Autodesk Fusion 360 part; units mm, degrees
(part 2 of 6)
  spline S358 degree 3 poles (-36.8879, 6.0923) (-36.784, 6.1608) (-36.7137, 6.2296) (-36.6303, 6.3216) knots 0 0 0 0 1 1 1 1
  spline S359 degree 3 poles (-36.6303, 6.3216) (-35.9723, 7.0157) (-35.2211, 7.6265) (-34.5007, 8.2547) knots 0 0 0 0 1 1 1 1
  spline S360 degree 3 poles (-34.5007, 8.2547) (-33.785, 8.879) (-33.0973, 9.5191) (-32.4627, 10.2268) knots 0 0 0 0 1 1 1 1
  spline S361 degree 3 poles (-32.4627, 10.2268) (-32.4451, 10.2088) (-32.4274, 10.1908) (-32.4092, 10.1722) knots 0 0 0 0 1 1 1 1
  spline S362 degree 3 poles (-32.4092, 10.1722) (-32.0575, 9.8145) (-31.7032, 9.4616) (-31.3264, 9.1303) knots 0 0 0 0 1 1 1 1
  spline S363 degree 3 poles (-31.3264, 9.1303) (-31.1837, 9.0046) (-31.0471, 8.8776) (-30.9171, 8.7388) knots 0 0 0 0 1 1 1 1
  spline S364 degree 3 poles (-30.9171, 8.7388) (-30.5101, 8.3132) (-30.1527, 8.1968) (-29.574, 8.1338) knots 0 0 0 0 1 1 1 1
  spline S365 degree 3 poles (-29.574, 8.1338) (-29.5084, 8.1252) (-29.4428, 8.1165) (-29.3772, 8.1077) knots 0 0 0 0 1 1 1 1
  spline S366 degree 3 poles (-29.3772, 8.1077) (-28.6438, 8.0188) (-27.9174, 8.0735) (-27.1848, 8.142) knots 0 0 0 0 1 1 1 1
  spline S367 degree 3 poles (-27.1848, 8.142) (-27.0333, 8.1561) (-26.8818, 8.17) (-26.7303, 8.1834) knots 0 0 0 0 1 1 1 1
  spline S368 degree 3 poles (-26.7303, 8.1834) (-26.6934, 8.1868) (-26.6565, 8.1901) (-26.6185, 8.1935) knots 0 0 0 0 1 1 1 1
  spline S369 degree 3 poles (-26.6185, 8.1935) (-26.3222, 8.2187) (-26.0268, 8.2275) (-25.7295, 8.224) knots 0 0 0 0 1 1 1 1
  spline S370 degree 3 poles (-25.7295, 8.224) (-25.4397, 8.2252) (-25.2695, 8.3218) (-25.0565, 8.5173) knots 0 0 0 0 1 1 1 1
  spline S371 degree 3 poles (-25.0565, 8.5173) (-24.9242, 8.5999) (-24.8512, 8.6377) (-24.6958, 8.6532) knots 0 0 0 0 1 1 1 1
  spline S372 degree 3 poles (-24.6958, 8.6532) (-24.4841, 8.7055) (-24.3698, 8.8291) (-24.2316, 8.9932) knots 0 0 0 0 1 1 1 1
  spline S373 degree 3 poles (-24.2316, 8.9932) (-24.1195, 9.1809) (-24.1288, 9.3727) (-24.1703, 9.5823) knots 0 0 0 0 1 1 1 1
  spline S374 degree 3 poles (-24.1703, 9.5823) (-24.2817, 9.9169) (-24.5269, 10.198) (-24.7398, 10.4737) knots 0 0 0 0 1 1 1 1
  spline S375 degree 3 poles (-24.7398, 10.4737) (-24.7778, 10.5239) (-24.8146, 10.5749) (-24.8506, 10.6265) knots 0 0 0 0 1 1 1 1
  spline S376 degree 3 poles (-24.8506, 10.6265) (-25.0198, 10.8677) (-25.0198, 10.8677) (-25.1822, 10.9142) knots 0 0 0 0 1 1 1 1
  spline S377 degree 3 poles (-25.1822, 10.9142) (-25.4781, 11.0159) (-25.7069, 11.2146) (-25.9398, 11.4183) knots 0 0 0 0 1 1 1 1
  spline S378 degree 3 poles (-25.9398, 11.4183) (-25.5444, 11.2634) (-25.1618, 11.083) (-24.7776, 10.9027) knots 0 0 0 0 1 1 1 1
  spline S379 degree 3 poles (-24.7776, 10.9027) (-24.4919, 10.7687) (-24.2046, 10.638) (-23.9172, 10.5075) knots 0 0 0 0 1 1 1 1
  spline S380 degree 3 poles (-23.9172, 10.5075) (-23.8009, 10.4547) (-23.6847, 10.4016) (-23.5685, 10.3486) knots 0 0 0 0 1 1 1 1
  spline S381 degree 3 poles (-23.5685, 10.3486) (-23.3419, 10.2452) (-23.1153, 10.142) (-22.8884, 10.0394) knots 0 0 0 0 1 1 1 1
  spline S382 degree 3 poles (-22.8884, 10.0394) (-22.8505, 10.0223) (-22.8126, 10.0051) (-22.7735, 9.9874) knots 0 0 0 0 1 1 1 1
  spline S383 degree 3 poles (-22.7735, 9.9874) (-22.7002, 9.9543) (-22.627, 9.9212) (-22.5537, 9.8881) knots 0 0 0 0 1 1 1 1
  spline S384 degree 3 poles (-22.5537, 9.8881) (-22.503, 9.8652) (-22.503, 9.8652) (-22.4513, 9.8418) knots 0 0 0 0 1 1 1 1
  spline S385 degree 3 poles (-22.4513, 9.8418) (-22.4218, 9.8285) (-22.3923, 9.8152) (-22.3619, 9.8015) knots 0 0 0 0 1 1 1 1
  spline S386 degree 3 poles (-22.3619, 9.8015) (-22.3034, 9.7745) (-22.2453, 9.7467) (-22.1885, 9.7163) knots 0 0 0 0 1 1 1 1
  spline S387 degree 3 poles (-22.1885, 9.7163) (-21.9936, 9.6149) (-21.8307, 9.5775) (-21.6123, 9.5674) knots 0 0 0 0 1 1 1 1
  spline S388 degree 3 poles (-21.6123, 9.5674) (-21.5658, 9.5644) (-21.5658, 9.5644) (-21.5185, 9.5615) knots 0 0 0 0 1 1 1 1
  spline S389 degree 3 poles (-21.5185, 9.5615) (-21.4183, 9.5554) (-21.3182, 9.5503) (-21.218, 9.5452) knots 0 0 0 0 1 1 1 1
  spline S390 degree 3 poles (-21.218, 9.5452) (-21.1484, 9.5413) (-21.0788, 9.5374) (-21.0092, 9.5334) knots 0 0 0 0 1 1 1 1
  spline S391 degree 3 poles (-21.0092, 9.5334) (-20.4466, 9.5024) (-19.8842, 9.482) (-19.3206, 9.4874) knots 0 0 0 0 1 1 1 1
  spline S392 degree 3 poles (-19.3206, 9.4874) (-19.2891, 9.4876) (-19.2575, 9.4878) (-19.225, 9.488) knots 0 0 0 0 1 1 1 1
  spline S393 degree 3 poles (-19.225, 9.488) (-18.1292, 9.5018) (-16.7384, 9.7508) (-15.913, 10.5426) knots 0 0 0 0 1 1 1 1
  spline S394 degree 3 poles (-15.913, 10.5426) (-15.7382, 10.7656) (-15.6089, 11.0119) (-15.6224, 11.3025) knots 0 0 0 0 1 1 1 1
  spline S395 degree 3 poles (-15.6224, 11.3025) (-15.6863, 11.7846) (-16.0023, 12.0234) (-16.3668, 12.3103) knots 0 0 0 0 1 1 1 1
  spline S396 degree 3 poles (-16.3668, 12.3103) (-16.8909, 12.6992) (-17.4415, 12.8815) (-18.0684, 13.0434) knots 0 0 0 0 1 1 1 1
  spline S397 degree 3 poles (-18.0684, 13.0434) (-18.3707, 13.1253) (-18.6252, 13.2381) (-18.8935, 13.3979) knots 0 0 0 0 1 1 1 1
  spline S398 degree 3 poles (-18.8935, 13.3979) (-19.3521, 13.6695) (-19.8084, 13.7489) (-20.3289, 13.6199) knots 0 0 0 0 1 1 1 1
  spline S399 degree 3 poles (-20.3289, 13.6199) (-20.5709, 13.5372) (-20.7719, 13.3642) (-20.9673, 13.2038) knots 0 0 0 0 1 1 1 1
  spline S400 degree 3 poles (-20.9673, 13.2038) (-21.0003, 13.2287) (-21.0003, 13.2287) (-21.034, 13.2542) knots 0 0 0 0 1 1 1 1
  spline S401 degree 3 poles (-21.034, 13.2542) (-21.681, 13.7272) (-22.4516, 13.9242) (-23.232, 14.051) knots 0 0 0 0 1 1 1 1
  spline S402 degree 3 poles (-23.232, 14.051) (-23.9763, 14.1741) (-24.6236, 14.5053) (-25.27, 14.8822) knots 0 0 0 0 1 1 1 1
  spline S403 degree 3 poles (-25.27, 14.8822) (-25.294, 14.896) (-25.3179, 14.9098) (-25.3425, 14.9239) knots 0 0 0 0 1 1 1 1
  spline S404 degree 3 poles (-25.3425, 14.9239) (-25.9243, 15.2588) (-26.4859, 15.6239) (-27.0332, 16.0126) knots 0 0 0 0 1 1 1 1
  spline S405 degree 3 poles (-27.0332, 16.0126) (-27.1228, 16.0743) (-27.2132, 16.1308) (-27.3071, 16.1857) knots 0 0 0 0 1 1 1 1
  spline S406 degree 3 poles (-27.3071, 16.1857) (-27.4896, 16.2931) (-27.661, 16.4146) (-27.8337, 16.5369) knots 0 0 0 0 1 1 1 1
  spline S407 degree 3 poles (-27.8337, 16.5369) (-28.0321, 16.6772) (-28.2298, 16.8138) (-28.4401, 16.9359) knots 0 0 0 0 1 1 1 1
  spline S408 degree 3 poles (-28.4401, 16.9359) (-28.5356, 16.993) (-28.6281, 17.0538) (-28.7209, 17.1152) knots 0 0 0 0 1 1 1 1
  spline S409 degree 3 poles (-28.7209, 17.1152) (-29.3537, 17.5298) (-30.124, 18.008) (-30.9074, 17.8632) knots 0 0 0 0 1 1 1 1
  spline S410 degree 3 poles (-30.9074, 17.8632) (-31.0398, 17.8256) (-31.1407, 17.7437) (-31.2552, 17.6685) knots 0 0 0 0 1 1 1 1
  spline S411 degree 3 poles (-31.2552, 17.6685) (-31.3254, 17.648) (-31.3962, 17.6296) (-31.4674, 17.613) knots 0 0 0 0 1 1 1 1
  spline S412 degree 3 poles (-31.4674, 17.613) (-31.8172, 17.5249) (-32.0335, 17.3244) (-32.2801, 17.0698) knots 0 0 0 0 1 1 1 1
  spline S413 degree 3 poles (-32.2801, 17.0698) (-32.3791, 16.9688) (-32.481, 16.8718) (-32.5848, 16.7757) knots 0 0 0 0 1 1 1 1
  spline S414 degree 3 poles (-32.5848, 16.7757) (-32.617, 16.7458) (-32.6492, 16.7159) (-32.6824, 16.685) knots 0 0 0 0 1 1 1 1
  spline S415 degree 3 poles (-32.6824, 16.685) (-32.7566, 16.6121) (-32.7566, 16.6121) (-32.8436, 16.6035) knots 0 0 0 0 1 1 1 1
  spline S416 degree 3 poles (-32.8436, 16.6035) (-32.8609, 16.6312) (-32.8782, 16.6588) (-32.896, 16.6872) knots 0 0 0 0 1 1 1 1
  spline S417 degree 3 poles (-32.896, 16.6872) (-33.2135, 17.1932) (-33.534, 17.6965) (-33.8742, 18.1877) knots 0 0 0 0 1 1 1 1
  spline S418 degree 3 poles (-33.8742, 18.1877) (-33.8992, 18.2239) (-33.9241, 18.2601) (-33.9498, 18.2975) knots 0 0 0 0 1 1 1 1
  spline S419 degree 3 poles (-33.9498, 18.2975) (-34.064, 18.4608) (-34.1797, 18.6215) (-34.3055, 18.7762) knots 0 0 0 0 1 1 1 1
  spline S420 degree 3 poles (-34.3055, 18.7762) (-34.6205, 19.1647) (-34.8641, 19.5705) (-35.0993, 20.0112) knots 0 0 0 0 1 1 1 1
  spline S421 degree 3 poles (-35.0993, 20.0112) (-35.5267, 20.8108) (-36.0105, 21.6081) (-36.9172, 21.9228) knots 0 0 0 0 1 1 1 1
  spline S422 degree 3 poles (-36.9172, 21.9228) (-37.0913, 21.9594) (-37.2565, 21.9237) (-37.4289, 21.8904) knots 0 0 0 0 1 1 1 1
  spline S423 degree 3 poles (-37.4289, 21.8904) (-37.4678, 21.8831) (-37.5066, 21.8758) (-37.5466, 21.8683) knots 0 0 0 0 1 1 1 1
  spline S424 degree 3 poles (-37.5466, 21.8683) (-38.3823, 21.6952) (-38.9884, 21.1445) (-39.5214, 20.5068) knots 0 0 0 0 1 1 1 1
  spline S425 degree 3 poles (-39.5214, 20.5068) (-39.5486, 20.4751) (-39.5758, 20.4434) (-39.6038, 20.4107) knots 0 0 0 0 1 1 1 1
  spline S426 degree 3 poles (-39.6038, 20.4107) (-39.7638, 20.2192) (-39.8932, 20.0166) (-40.0164, 19.8) knots 0 0 0 0 1 1 1 1
  spline S427 degree 3 poles (-40.0164, 19.8) (-40.0388, 19.7605) (-40.0612, 19.7211) (-40.0844, 19.6805) knots 0 0 0 0 1 1 1 1
  spline S428 degree 3 poles (-40.0844, 19.6805) (-40.1778, 19.515) (-40.2706, 19.3492) (-40.3602, 19.1815) knots 0 0 0 0 1 1 1 1
  spline S429 degree 3 poles (-40.3602, 19.1815) (-40.5125, 18.8967) (-40.6813, 18.6249) (-40.8569, 18.3542) knots 0 0 0 0 1 1 1 1
  spline S430 degree 3 poles (-40.8569, 18.3542) (-40.923, 18.2523) (-40.9887, 18.1501) (-41.0544, 18.048) knots 0 0 0 0 1 1 1 1
  spline S431 degree 3 poles (-41.0544, 18.048) (-41.0856, 17.9994) (-41.1169, 17.9508) (-41.1482, 17.9023) knots 0 0 0 0 1 1 1 1
  spline S432 degree 3 poles (-41.1482, 17.9023) (-41.179, 17.8545) (-41.2097, 17.8066) (-41.2402, 17.7586) knots 0 0 0 0 1 1 1 1
  spline S433 degree 3 poles (-41.2402, 17.7586) (-41.2802, 17.6959) (-41.3208, 17.6336) (-41.3616, 17.5714) knots 0 0 0 0 1 1 1 1
  spline S434 degree 3 poles (-41.3616, 17.5714) (-41.5465, 17.2846) (-41.6929, 16.9906) (-41.8309, 16.6789) knots 0 0 0 0 1 1 1 1
  spline S435 degree 3 poles (-41.8309, 16.6789) (-42.0704, 16.1135) (-42.0704, 16.1135) (-42.5077, 15.6951) knots 0 0 0 0 1 1 1 1
  spline S436 degree 3 poles (-42.5077, 15.6951) (-42.6276, 15.6587) (-42.7094, 15.6838) (-42.8309, 15.7125) knots 0 0 0 0 1 1 1 1
  spline S437 degree 3 poles (-42.8309, 15.7125) (-42.8779, 15.7234) (-42.9248, 15.7343) (-42.9731, 15.7456) knots 0 0 0 0 1 1 1 1
  spline S438 degree 3 poles (-42.9731, 15.7456) (-43.0476, 15.7637) (-43.0476, 15.7637) (-43.1237, 15.7823) knots 0 0 0 0 1 1 1 1
  spline S439 degree 3 poles (-43.1237, 15.7823) (-43.1743, 15.7942) (-43.2249, 15.8061) (-43.277, 15.8184) knots 0 0 0 0 1 1 1 1
  spline S440 degree 3 poles (-43.277, 15.8184) (-43.5852, 15.892) (-43.888, 15.9728) (-44.1875, 16.0763) knots 0 0 0 0 1 1 1 1
  spline S441 degree 3 poles (-44.1875, 16.0763) (-44.3054, 16.104) (-44.3939, 16.111) (-44.5135, 16.111) knots 0 0 0 0 1 1 1 1
  spline S442 degree 3 poles (-44.5135, 16.111) (-44.7686, 16.1124) (-45.0072, 16.166) (-45.2558, 16.2195) knots 0 0 0 0 1 1 1 1
  spline S443 degree 3 poles (-45.2558, 16.2195) (-46.3261, 16.4374) (-47.3716, 16.5413) (-48.4437, 16.2899) knots 0 0 0 0 1 1 1 1
  spline S444 degree 3 poles (-48.4437, 16.2899) (-48.4742, 16.2832) (-48.5047, 16.2765) (-48.5362, 16.2696) knots 0 0 0 0 1 1 1 1
  spline S445 degree 3 poles (-48.5362, 16.2696) (-49.2063, 16.1143) (-49.7697, 15.7409) (-50.344, 15.3773) knots 0 0 0 0 1 1 1 1
  spline S446 degree 3 poles (-50.344, 15.3773) (-50.4556, 15.307) (-50.5645, 15.241) (-50.6872, 15.1921) knots 0 0 0 0 1 1 1 1
  spline S447 degree 3 poles (-50.6872, 15.1921) (-50.6691, 15.2109) (-50.651, 15.2297) (-50.6323, 15.2491) knots 0 0 0 0 1 1 1 1
  spline S448 degree 3 poles (-50.6323, 15.2491) (-50.4501, 15.4534) (-50.3811, 15.6233) (-50.3221, 15.8884) knots 0 0 0 0 1 1 1 1
  spline S449 degree 3 poles (-50.3221, 15.8884) (-50.1794, 16.4731) (-49.682, 16.8133) (-49.2179, 17.1446) knots 0 0 0 0 1 1 1 1
  spline S450 degree 3 poles (-49.2179, 17.1446) (-49.0182, 17.2877) (-48.8217, 17.435) (-48.6251, 17.5823) knots 0 0 0 0 1 1 1 1
  spline S451 degree 3 poles (-48.6251, 17.5823) (-48.5603, 17.6304) (-48.4948, 17.6776) (-48.4293, 17.7247) knots 0 0 0 0 1 1 1 1
  spline S452 degree 3 poles (-48.4293, 17.7247) (-48.0216, 18.0274) (-47.557, 18.5172) (-47.4394, 19.0281) knots 0 0 0 0 1 1 1 1
  spline S453 degree 3 poles (-47.4394, 19.0281) (-47.463, 19.2434) (-47.4932, 19.4392) (-47.6255, 19.6149) knots 0 0 0 0 1 1 1 1
  spline S454 degree 3 poles (-47.6255, 19.6149) (-48.0279, 19.8024) (-48.4467, 19.7521) (-48.8536, 19.61) knots 0 0 0 0 1 1 1 1
  spline S455 degree 3 poles (-48.8536, 19.61) (-49.2499, 19.4463) (-49.6121, 19.2138) (-49.9763, 18.9893) knots 0 0 0 0 1 1 1 1
  spline S456 degree 3 poles (-49.9763, 18.9893) (-50.2765, 18.8143) (-50.6627, 18.7282) (-51.0047, 18.8097) knots 0 0 0 0 1 1 1 1
  spline S457 degree 3 poles (-51.0047, 18.8097) (-51.0936, 18.8443) (-51.1659, 18.8904) (-51.2454, 18.943) knots 0 0 0 0 1 1 1 1
  spline S458 degree 3 poles (-51.2454, 18.943) (-51.389, 19.034) (-51.4771, 19.0454) (-51.6426, 19.014) knots 0 0 0 0 1 1 1 1
  spline S459 degree 3 poles (-51.6426, 19.014) (-51.7259, 18.9745) (-51.7259, 18.9745) (-51.8388, 18.8732) knots 0 0 0 0 1 1 1 1
  spline S460 degree 3 poles (-51.8388, 18.8732) (-51.9741, 18.7595) (-52.1019, 18.7139) (-52.2735, 18.6677) knots 0 0 0 0 1 1 1 1
  spline S461 degree 3 poles (-52.2735, 18.6677) (-52.331, 18.6516) (-52.3884, 18.6356) (-52.4459, 18.6195) knots 0 0 0 0 1 1 1 1
  spline S462 degree 3 poles (-52.4459, 18.6195) (-52.4756, 18.6115) (-52.5054, 18.6034) (-52.536, 18.5951) knots 0 0 0 0 1 1 1 1
  spline S463 degree 3 poles (-52.536, 18.5951) (-53.1106, 18.439) (-53.6573, 18.2525) (-54.198, 18.0016) knots 0 0 0 0 1 1 1 1
  spline S464 degree 3 poles (-54.198, 18.0016) (-54.6047, 17.814) (-55.0066, 17.6569) (-55.4376, 17.5352) knots 0 0 0 0 1 1 1 1
  spline S465 degree 3 poles (-55.4376, 17.5352) (-55.4604, 17.5687) (-55.4604, 17.5687) (-55.4836, 17.6029) knots 0 0 0 0 1 1 1 1
  spline S466 degree 3 poles (-55.4836, 17.6029) (-55.6209, 17.7753) (-55.8226, 17.8559) (-56.0361, 17.884) knots 0 0 0 0 1 1 1 1
  spline S467 degree 3 poles (-56.0361, 17.884) (-56.1445, 17.8761) (-56.2456, 17.8642) (-56.3522, 17.8463) knots 0 0 0 0 1 1 1 1
  spline S468 degree 3 poles (-56.3522, 17.8463) (-56.3919, 17.8414) (-56.3919, 17.8414) (-56.4323, 17.8363) knots 0 0 0 0 1 1 1 1
  spline S469 degree 3 poles (-56.4323, 17.8363) (-57.0096, 17.7406) (-57.5367, 17.3205) (-58.0104, 16.9992) knots 0 0 0 0 1 1 1 1
  spline S470 degree 3 poles (-58.0104, 16.9992) (-58.3797, 16.7497) (-58.7477, 16.5551) (-59.1587, 16.3833) knots 0 0 0 0 1 1 1 1
  spline S471 degree 3 poles (-59.1587, 16.3833) (-59.2277, 16.3521) (-59.2965, 16.3206) (-59.3651, 16.2885) knots 0 0 0 0 1 1 1 1
  spline S472 degree 3 poles (-59.3651, 16.2885) (-59.3944, 16.275) (-59.4236, 16.2614) (-59.4537, 16.2474) knots 0 0 0 0 1 1 1 1
  spline S473 degree 3 poles (-59.4537, 16.2474) (-59.5111, 16.2206) (-59.5686, 16.1938) (-59.626, 16.167) knots 0 0 0 0 1 1 1 1
  spline S474 degree 3 poles (-59.626, 16.167) (-59.6549, 16.1536) (-59.6837, 16.1402) (-59.7135, 16.1264) knots 0 0 0 0 1 1 1 1
  spline S475 degree 3 poles (-59.7135, 16.1264) (-59.7417, 16.1133) (-59.7699, 16.1002) (-59.7989, 16.0867) knots 0 0 0 0 1 1 1 1
  spline S476 degree 3 poles (-59.7989, 16.0867) (-59.8853, 16.0485) (-59.9727, 16.015) (-60.0609, 15.9812) knots 0 0 0 0 1 1 1 1
  spline S477 degree 3 poles (-60.0609, 15.9812) (-60.2413, 15.907) (-60.3774, 15.8013) (-60.5265, 15.6775) knots 0 0 0 0 1 1 1 1
  spline S478 degree 3 poles (-60.5265, 15.6775) (-60.8228, 15.4401) (-61.1293, 15.22) (-61.4422, 15.0053) knots 0 0 0 0 1 1 1 1
  spline S479 degree 3 poles (-61.4422, 15.0053) (-61.4931, 14.9704) (-61.544, 14.9352) (-61.5948, 14.9) knots 0 0 0 0 1 1 1 1
  spline S480 degree 3 poles (-61.5948, 14.9) (-61.667, 14.85) (-61.7395, 14.8004) (-61.8121, 14.751) knots 0 0 0 0 1 1 1 1
  spline S481 degree 3 poles (-61.8121, 14.751) (-61.8541, 14.7222) (-61.8962, 14.6934) (-61.9395, 14.6637) knots 0 0 0 0 1 1 1 1
  spline S482 degree 3 poles (-61.9395, 14.6637) (-62.1493, 14.5407) (-62.3244, 14.4856) (-62.5654, 14.5176) knots 0 0 0 0 1 1 1 1
  spline S483 degree 3 poles (-62.5654, 14.5176) (-63.3565, 14.5876) (-64.0549, 14.3462) (-64.6704, 13.8507) knots 0 0 0 0 1 1 1 1
  spline S484 degree 3 poles (-64.6704, 13.8507) (-64.9868, 13.5794) (-65.2483, 13.2746) (-65.5102, 12.952) knots 0 0 0 0 1 1 1 1
  spline S485 degree 3 poles (-65.5102, 12.952) (-65.5405, 12.9147) (-65.5405, 12.9147) (-65.5715, 12.8767) knots 0 0 0 0 1 1 1 1
  spline S486 degree 3 poles (-65.5715, 12.8767) (-65.6101, 12.8292) (-65.6485, 12.7816) (-65.6867, 12.7337) knots 0 0 0 0 1 1 1 1
  spline S487 degree 3 poles (-65.6867, 12.7337) (-66.0286, 12.3111) (-66.4249, 11.9667) (-66.8463, 11.6259) knots 0 0 0 0 1 1 1 1
  spline S488 degree 3 poles (-66.8463, 11.6259) (-67.102, 11.4159) (-67.3243, 11.1965) (-67.5345, 10.941) knots 0 0 0 0 1 1 1 1
  spline S489 degree 3 poles (-67.5345, 10.941) (-67.5595, 10.9112) (-67.5845, 10.8815) (-67.6103, 10.8508) knots 0 0 0 0 1 1 1 1
  spline S490 degree 3 poles (-67.6103, 10.8508) (-68.0141, 10.3567) (-68.1173, 9.5556) (-68.0597, 8.9377) knots 0 0 0 0 1 1 1 1
  spline S491 degree 3 poles (-68.0597, 8.9377) (-67.8934, 7.6051) (-67.2744, 6.568) (-66.5667, 5.4526) knots 0 0 0 0 1 1 1 1
  spline S492 degree 3 poles (-66.5667, 5.4526) (-66.5415, 5.4125) (-66.5163, 5.3724) (-66.4904, 5.3311) knots 0 0 0 0 1 1 1 1
  spline S493 degree 3 poles (-66.4904, 5.3311) (-66.4655, 5.2916) (-66.4405, 5.2522) (-66.4148, 5.2115) knots 0 0 0 0 1 1 1 1
  spline S494 degree 3 poles (-66.4148, 5.2115) (-66.3924, 5.1759) (-66.37, 5.1403) (-66.3468, 5.1036) knots 0 0 0 0 1 1 1 1
  spline S495 degree 3 poles (-66.3468, 5.1036) (-66.1436, 4.8029) (-65.891, 4.673) (-65.5627, 4.5317) knots 0 0 0 0 1 1 1 1
  spline S496 degree 3 poles (-65.5627, 4.5317) (-65.4217, 4.4709) (-65.2852, 4.4033) (-65.1485, 4.3335) knots 0 0 0 0 1 1 1 1
  spline S497 degree 3 poles (-65.1485, 4.3335) (-64.5048, 4.0056) (-63.893, 3.8018) (-63.1622, 3.8179) knots 0 0 0 0 1 1 1 1
  spline S498 degree 3 poles (-63.1622, 3.8179) (-63.0974, 3.8188) (-63.0974, 3.8188) (-63.0313, 3.8198) knots 0 0 0 0 1 1 1 1
  spline S499 degree 3 poles (-63.0313, 3.8198) (-62.9408, 3.8211) (-62.8502, 3.8227) (-62.7596, 3.8245) knots 0 0 0 0 1 1 1 1
  spline S500 degree 3 poles (-62.7596, 3.8245) (-62.622, 3.8272) (-62.4844, 3.8293) (-62.3467, 3.8313) knots 0 0 0 0 1 1 1 1
  spline S501 degree 3 poles (-62.3467, 3.8313) (-62.2582, 3.8327) (-62.1696, 3.8341) (-62.081, 3.8356) knots 0 0 0 0 1 1 1 1
  spline S502 degree 3 poles (-62.081, 3.8356) (-62.0201, 3.8366) (-62.0201, 3.8366) (-61.958, 3.8376) knots 0 0 0 0 1 1 1 1
  spline S503 degree 3 poles (-61.958, 3.8376) (-60.1229, 3.8743) (-58.2945, 4.4626) (-56.8097, 5.5496) knots 0 0 0 0 1 1 1 1
  spline S504 degree 3 poles (-56.8097, 5.5496) (-56.6794, 5.6468) (-56.6794, 5.6468) (-56.5257, 5.6878) knots 0 0 0 0 1 1 1 1
  spline S505 degree 3 poles (-56.5257, 5.6878) (-56.439, 5.6747) (-56.439, 5.6747) (-56.3829, 5.6059) knots 0 0 0 0 1 1 1 1
  spline S506 degree 3 poles (-56.3829, 5.6059) (-56.2885, 5.4409) (-56.2394, 5.2593) (-56.1818, 5.0789) knots 0 0 0 0 1 1 1 1
  spline S507 degree 3 poles (-56.1818, 5.0789) (-56.1663, 5.031) (-56.1509, 4.983) (-56.1349, 4.9336) knots 0 0 0 0 1 1 1 1
  spline S508 degree 3 poles (-56.1349, 4.9336) (-55.9815, 4.4497) (-55.8516, 3.9594) (-55.7199, 3.4693) knots 0 0 0 0 1 1 1 1
  spline S509 degree 3 poles (-55.7199, 3.4693) (-55.1814, 1.4664) (-54.5799, -0.5857) (-52.7021, -1.7273) knots 0 0 0 0 1 1 1 1
  spline S510 degree 3 poles (-52.7021, -1.7273) (-52.1368, -2.0407) (-52.1368, -2.0407) (-51.9904, -2.0149) knots 0 0 0 0 1 1 1 1
  spline S511 degree 3 poles (-51.9904, -2.0149) (-51.9906, -2.0524) (-51.9908, -2.0899) (-51.991, -2.1286) knots 0 0 0 0 1 1 1 1
  spline S512 degree 3 poles (-51.991, -2.1286) (-51.9636, -2.8299) (-51.645, -3.4042) (-51.3097, -4.0015) knots 0 0 0 0 1 1 1 1
  spline S513 degree 3 poles (-51.3097, -4.0015) (-51.3453, -4.0094) (-51.3453, -4.0094) (-51.3816, -4.0174) knots 0 0 0 0 1 1 1 1
  spline S514 degree 3 poles (-51.3816, -4.0174) (-52.0739, -4.1867) (-52.7152, -4.5109) (-53.2315, -5.0035) knots 0 0 0 0 1 1 1 1
  spline S515 degree 3 poles (-53.2315, -5.0035) (-53.3705, -5.1323) (-53.4674, -5.2003) (-53.6593, -5.2006) knots 0 0 0 0 1 1 1 1
  spline S516 degree 3 poles (-53.6593, -5.2006) (-53.7599, -5.1657) (-53.8483, -5.129) (-53.9434, -5.0829) knots 0 0 0 0 1 1 1 1
  spline S517 degree 3 poles (-53.9434, -5.0829) (-55.9004, -4.2074) (-58.0187, -5.0468) (-59.9027, -5.7123) knots 0 0 0 0 1 1 1 1
  spline S518 degree 3 poles (-59.9027, -5.7123) (-60.2035, -5.8184) (-60.5051, -5.9214) (-60.8077, -6.0222) knots 0 0 0 0 1 1 1 1
  spline S519 degree 3 poles (-60.8077, -6.0222) (-60.8482, -6.0358) (-60.8886, -6.0493) (-60.9303, -6.0633) knots 0 0 0 0 1 1 1 1
  spline S520 degree 3 poles (-60.9303, -6.0633) (-61.0381, -6.099) (-61.1461, -6.1339) (-61.2544, -6.1681) knots 0 0 0 0 1 1 1 1
  spline S521 degree 3 poles (-61.2544, -6.1681) (-61.2996, -6.1825) (-61.2996, -6.1825) (-61.3456, -6.1972) knots 0 0 0 0 1 1 1 1
  spline S522 degree 3 poles (-61.3456, -6.1972) (-61.6363, -6.2846) (-61.934, -6.3369) (-62.2324, -6.3895) knots 0 0 0 0 1 1 1 1
  spline S523 degree 3 poles (-62.2324, -6.3895) (-62.3222, -6.4054) (-62.4119, -6.422) (-62.5016, -6.4386) knots 0 0 0 0 1 1 1 1
  spline S524 degree 3 poles (-62.5016, -6.4386) (-63.1944, -6.5706) (-63.1944, -6.5706) (-63.8495, -6.3701) knots 0 0 0 0 1 1 1 1
  spline S525 degree 3 poles (-63.8495, -6.3701) (-63.8786, -6.3546) (-63.9077, -6.339) (-63.9377, -6.323) knots 0 0 0 0 1 1 1 1
  spline S526 degree 3 poles (-63.9377, -6.323) (-63.9949, -6.2924) (-64.0519, -6.2614) (-64.1086, -6.2299) knots 0 0 0 0 1 1 1 1
  spline S527 degree 3 poles (-64.1086, -6.2299) (-64.1998, -6.18) (-64.2933, -6.1357) (-64.3868, -6.0905) knots 0 0 0 0 1 1 1 1
  spline S528 degree 3 poles (-64.3868, -6.0905) (-64.5845, -5.986) (-64.761, -5.8541) (-64.942, -5.7237) knots 0 0 0 0 1 1 1 1
  spline S529 degree 3 poles (-64.942, -5.7237) (-65.255, -5.4989) (-65.5487, -5.3398) (-65.9234, -5.2384) knots 0 0 0 0 1 1 1 1
  spline S530 degree 3 poles (-65.9234, -5.2384) (-66.0477, -5.198) (-66.1425, -5.1475) (-66.2555, -5.0827) knots 0 0 0 0 1 1 1 1
  spline S531 degree 3 poles (-66.2555, -5.0827) (-67.2908, -4.5046) (-68.5469, -4.3059) (-69.7187, -4.3147) knots 0 0 0 0 1 1 1 1
  spline S532 degree 3 poles (-69.7187, -4.3147) (-69.7712, -4.3147) (-69.8237, -4.3147) (-69.8778, -4.3147) knots 0 0 0 0 1 1 1 1
  spline S533 degree 3 poles (-69.8778, -4.3147) (-70.2207, -4.3231) (-70.5539, -4.37) (-70.8918, -4.426) knots 0 0 0 0 1 1 1 1
  spline S534 degree 3 poles (-70.8918, -4.426) (-70.9339, -4.4327) (-70.9759, -4.4394) (-71.0192, -4.4463) knots 0 0 0 0 1 1 1 1
  spline S535 degree 3 poles (-71.0192, -4.4463) (-71.5269, -4.5363) (-71.9207, -4.7633) (-72.2275, -5.1851) knots 0 0 0 0 1 1 1 1
  spline S536 degree 3 poles (-72.2275, -5.1851) (-72.3637, -5.399) (-72.4828, -5.6214) (-72.5986, -5.8468) knots 0 0 0 0 1 1 1 1
  spline S537 degree 3 poles (-72.5986, -5.8468) (-72.6546, -5.9506) (-72.7163, -6.0487) (-72.7801, -6.1479) knots 0 0 0 0 1 1 1 1
  spline S538 degree 3 poles (-72.7801, -6.1479) (-72.9035, -6.3449) (-72.9941, -6.549) (-73.0848, -6.7625) knots 0 0 0 0 1 1 1 1
  spline S539 degree 3 poles (-73.0848, -6.7625) (-73.2634, -7.1723) (-73.4816, -7.563) (-73.7041, -7.9502) knots 0 0 0 0 1 1 1 1
  spline S540 degree 3 poles (-73.7041, -7.9502) (-73.7179, -7.9743) (-73.7316, -7.9983) (-73.7458, -8.023) knots 0 0 0 0 1 1 1 1
  spline S541 degree 3 poles (-73.7458, -8.023) (-73.9174, -8.3215) (-74.0931, -8.6166) (-74.2768, -8.9079) knots 0 0 0 0 1 1 1 1
  spline S542 degree 3 poles (-74.2768, -8.9079) (-74.3558, -9.0336) (-74.4324, -9.1607) (-74.5089, -9.288) knots 0 0 0 0 1 1 1 1
  spline S543 degree 3 poles (-74.5089, -9.288) (-74.5741, -9.3949) (-74.6411, -9.5007) (-74.708, -9.6066) knots 0 0 0 0 1 1 1 1
  spline S544 degree 3 poles (-74.708, -9.6066) (-74.8384, -9.8136) (-74.9561, -10.0259) (-75.0703, -10.2421) knots 0 0 0 0 1 1 1 1
  spline S545 degree 3 poles (-75.0703, -10.2421) (-75.143, -10.3569) (-75.2065, -10.4303) (-75.3186, -10.5068) knots 0 0 0 0 1 1 1 1
  spline S546 degree 3 poles (-75.3186, -10.5068) (-75.4881, -10.5374) (-75.6201, -10.4209) (-75.755, -10.3308) knots 0 0 0 0 1 1 1 1
  spline S547 degree 3 poles (-75.755, -10.3308) (-75.7812, -10.3136) (-75.8075, -10.2965) (-75.8345, -10.2788) knots 0 0 0 0 1 1 1 1
  spline S548 degree 3 poles (-75.8345, -10.2788) (-76.0434, -10.1412) (-76.2473, -9.9967) (-76.4513, -9.852) knots 0 0 0 0 1 1 1 1
  spline S549 degree 3 poles (-76.4513, -9.852) (-76.7266, -9.6571) (-77.0027, -9.4835) (-77.3026, -9.3283) knots 0 0 0 0 1 1 1 1
  spline S550 degree 3 poles (-77.3026, -9.3283) (-77.3412, -9.3073) (-77.3798, -9.2863) (-77.4196, -9.2647) knots 0 0 0 0 1 1 1 1
  spline S551 degree 3 poles (-77.4196, -9.2647) (-78.1033, -8.9074) (-78.9925, -8.6536) (-79.7502, -8.8776) knots 0 0 0 0 1 1 1 1
  spline S552 degree 3 poles (-79.7502, -8.8776) (-79.9183, -8.9311) (-80.083, -8.9914) (-80.2475, -9.055) knots 0 0 0 0 1 1 1 1
  spline S553 degree 3 poles (-80.2475, -9.055) (-80.2801, -9.067) (-80.3128, -9.0791) (-80.3464, -9.0915) knots 0 0 0 0 1 1 1 1
  spline S554 degree 3 poles (-80.3464, -9.0915) (-80.6659, -9.2148) (-80.9042, -9.3674) (-81.0849, -9.6647) knots 0 0 0 0 1 1 1 1
  spline S555 degree 3 poles (-81.0849, -9.6647) (-81.1051, -9.6964) (-81.1254, -9.7281) (-81.1462, -9.7608) knots 0 0 0 0 1 1 1 1
  spline S556 degree 3 poles (-81.1462, -9.7608) (-81.231, -9.9376) (-81.2647, -10.1121) (-81.3, -10.3042) knots 0 0 0 0 1 1 1 1
  spline S557 degree 3 poles (-81.3, -10.3042) (-81.3073, -10.3437) (-81.3147, -10.3831) (-81.3223, -10.4238) knots 0 0 0 0 1 1 1 1
  spline S558 degree 3 poles (-81.3223, -10.4238) (-81.5295, -11.5933) (-81.5096, -12.9952) (-80.9381, -14.071) knots 0 0 0 0 1 1 1 1
  spline S559 degree 3 poles (-80.9381, -14.071) (-80.8732, -14.1963) (-80.8303, -14.2822) (-80.8599, -14.4236) knots 0 0 0 0 1 1 1 1
  spline S560 degree 3 poles (-80.8599, -14.4236) (-80.9019, -14.5264) (-80.9506, -14.6213) (-81.0044, -14.7184) knots 0 0 0 0 1 1 1 1
  spline S561 degree 3 poles (-81.0044, -14.7184) (-81.0227, -14.7536) (-81.041, -14.7887) (-81.0598, -14.825) knots 0 0 0 0 1 1 1 1
  spline S562 degree 3 poles (-81.0598, -14.825) (-81.2073, -15.1051) (-81.3656, -15.3796) (-81.5308, -15.6497) knots 0 0 0 0 1 1 1 1
  spline S563 degree 3 poles (-81.5308, -15.6497) (-81.5519, -15.6844) (-81.5519, -15.6844) (-81.5734, -15.7199) knots 0 0 0 0 1 1 1 1
  spline S564 degree 3 poles (-81.5734, -15.7199) (-81.6024, -15.7672) (-81.6322, -15.8141) (-81.6626, -15.8605) knots 0 0 0 0 1 1 1 1
  spline S565 degree 3 poles (-81.6626, -15.8605) (-81.818, -16.1078) (-81.7716, -16.2778) (-81.6891, -16.5457) knots 0 0 0 0 1 1 1 1
  spline S566 degree 3 poles (-61.3294, -20.2671) (-61.263, -20.2962) (-61.263, -20.2962) (-61.1951, -20.326) knots 0 0 0 0 1 1 1 1
  spline S567 degree 3 poles (-61.1951, -20.326) (-61.2348, -20.333) (-61.2744, -20.34) (-61.3153, -20.3472) knots 0 0 0 0 1 1 1 1
  spline S568 degree 3 poles (-61.3153, -20.3472) (-61.32, -20.3207) (-61.3246, -20.2943) (-61.3294, -20.2671) knots 0 0 0 0 1 1 1 1
  spline S569 degree 3 poles (-59.751, 10.372) (-59.6633, 10.465) (-59.5616, 10.5119) (-59.4464, 10.565) knots 0 0 0 0 1 1 1 1
  spline S570 degree 3 poles (-59.4464, 10.565) (-59.4153, 10.5807) (-59.3843, 10.5964) (-59.3523, 10.6127) knots 0 0 0 0 1 1 1 1
  spline S571 degree 3 poles (-59.3523, 10.6127) (-59.2858, 10.6462) (-59.219, 10.6791) (-59.152, 10.7115) knots 0 0 0 0 1 1 1 1
  spline S572 degree 3 poles (-59.152, 10.7115) (-58.977, 10.7962) (-58.8043, 10.8855) (-58.6312, 10.9741) knots 0 0 0 0 1 1 1 1
  spline S573 degree 3 poles (-58.6312, 10.9741) (-58.5971, 10.9914) (-58.5629, 11.0088) (-58.5277, 11.0266) knots 0 0 0 0 1 1 1 1
  spline S574 degree 3 poles (-58.5277, 11.0266) (-57.7705, 11.4124) (-57.0352, 11.9023) (-56.4295, 12.5015) knots 0 0 0 0 1 1 1 1
  spline S575 degree 3 poles (-56.4295, 12.5015) (-56.0056, 12.9201) (-55.4738, 13.0694) (-54.9102, 13.212) knots 0 0 0 0 1 1 1 1
  spline S576 degree 3 poles (-54.9102, 13.212) (-54.2791, 13.3732) (-53.6906, 13.592) (-53.0958, 13.8587) knots 0 0 0 0 1 1 1 1
  spline S577 degree 3 poles (-53.0958, 13.8587) (-52.9602, 13.9188) (-52.8245, 13.9787) (-52.6887, 14.0383) knots 0 0 0 0 1 1 1 1
  spline S578 degree 3 poles (-52.6887, 14.0383) (-52.6043, 14.0754) (-52.52, 14.113) (-52.4359, 14.151) knots 0 0 0 0 1 1 1 1
  spline S579 degree 3 poles (-52.4359, 14.151) (-52.3984, 14.1676) (-52.3609, 14.1843) (-52.3223, 14.2014) knots 0 0 0 0 1 1 1 1
  spline S580 degree 3 poles (-52.3223, 14.2014) (-52.2894, 14.2163) (-52.2565, 14.2311) (-52.2226, 14.2464) knots 0 0 0 0 1 1 1 1
  spline S581 degree 3 poles (-52.2226, 14.2464) (-52.1313, 14.2848) (-52.1313, 14.2848) (-52.0094, 14.2568) knots 0 0 0 0 1 1 1 1
  spline S582 degree 3 poles (-52.0094, 14.2568) (-52.0534, 14.2314) (-52.0974, 14.206) (-52.1428, 14.1798) knots 0 0 0 0 1 1 1 1
  spline S583 degree 3 poles (-52.1428, 14.1798) (-52.5791, 13.919) (-52.9072, 13.6269) (-53.2354, 13.2404) knots 0 0 0 0 1 1 1 1
  spline S584 degree 3 poles (-53.2354, 13.2404) (-53.3211, 13.1403) (-53.4099, 13.0432) (-53.4989, 12.946) knots 0 0 0 0 1 1 1 1
  spline S585 degree 3 poles (-53.4989, 12.946) (-53.6938, 12.7322) (-53.8771, 12.5123) (-54.0526, 12.2821) knots 0 0 0 0 1 1 1 1
  spline S586 degree 3 poles (-54.0526, 12.2821) (-54.1106, 12.2071) (-54.1701, 12.136) (-54.233, 12.0652) knots 0 0 0 0 1 1 1 1
  spline S587 degree 3 poles (-54.233, 12.0652) (-54.3312, 11.9443) (-54.4082, 11.8212) (-54.4872, 11.6874) knots 0 0 0 0 1 1 1 1
  spline S588 degree 3 poles (-54.4872, 11.6874) (-54.5654, 11.5559) (-54.6458, 11.4259) (-54.7274, 11.2965) knots 0 0 0 0 1 1 1 1
  spline S589 degree 3 poles (-54.7274, 11.2965) (-54.7428, 11.2721) (-54.7582, 11.2477) (-54.774, 11.2226) knots 0 0 0 0 1 1 1 1
  spline S590 degree 3 poles (-54.774, 11.2226) (-54.857, 11.093) (-54.9434, 10.9736) (-55.0452, 10.8584) knots 0 0 0 0 1 1 1 1
  spline S591 degree 3 poles (-55.0452, 10.8584) (-55.2359, 10.6313) (-55.3492, 10.3545) (-55.4744, 10.0881) knots 0 0 0 0 1 1 1 1
  spline S592 degree 3 poles (-55.4744, 10.0881) (-55.5326, 9.9644) (-55.5924, 9.8415) (-55.6523, 9.7187) knots 0 0 0 0 1 1 1 1
  spline S593 degree 3 poles (-55.6523, 9.7187) (-55.6804, 9.6603) (-55.6804, 9.6603) (-55.7091, 9.6007) knots 0 0 0 0 1 1 1 1
  spline S594 degree 3 poles (-55.7091, 9.6007) (-55.7555, 9.5039) (-55.7555, 9.5039) (-55.8229, 9.4123) knots 0 0 0 0 1 1 1 1
  spline S595 degree 3 poles (-55.8229, 9.4123) (-55.931, 9.3943) (-56.0328, 9.3834) (-56.1419, 9.3767) knots 0 0 0 0 1 1 1 1
  spline S596 degree 3 poles (-56.1419, 9.3767) (-56.1755, 9.3747) (-56.2092, 9.3726) (-56.2439, 9.3704) knots 0 0 0 0 1 1 1 1
  spline S597 degree 3 poles (-56.2439, 9.3704) (-56.9302, 9.336) (-57.6315, 9.3267) (-58.2906, 9.5376) knots 0 0 0 0 1 1 1 1
  spline S598 degree 3 poles (-58.2906, 9.5376) (-58.5865, 9.6318) (-58.8906, 9.6973) (-59.1928, 9.7682) knots 0 0 0 0 1 1 1 1
  spline S599 degree 3 poles (-59.1928, 9.7682) (-59.2522, 9.7823) (-59.3116, 9.7963) (-59.3711, 9.8104) knots 0 0 0 0 1 1 1 1
  spline S600 degree 3 poles (-59.3711, 9.8104) (-59.5119, 9.8438) (-59.6527, 9.877) (-59.7935, 9.9101) knots 0 0 0 0 1 1 1 1
  spline S601 degree 3 poles (-59.7935, 9.9101) (-59.8214, 10.0683) (-59.8022, 10.2204) (-59.751, 10.372) knots 0 0 0 0 1 1 1 1
  spline S602 degree 3 poles (-50.3728, -11.189) (-49.7763, -10.9024) (-49.2643, -10.7643) (-48.6006, -10.8145) knots 0 0 0 0 1 1 1 1
  spline S603 degree 3 poles (-48.6006, -10.8145) (-47.8499, -10.8686) (-47.154, -10.6753) (-46.4412, -10.4578) knots 0 0 0 0 1 1 1 1
  spline S604 degree 3 poles (-46.4412, -10.4578) (-45.8156, -10.2684) (-45.2693, -10.1602) (-44.6228, -10.299) knots 0 0 0 0 1 1 1 1
  spline S605 degree 3 poles (-44.6228, -10.299) (-44.6249, -10.4252) (-44.6279, -10.5513) (-44.631, -10.6774) knots 0 0 0 0 1 1 1 1
  spline S606 degree 3 poles (-44.631, -10.6774) (-44.6318, -10.7306) (-44.6318, -10.7306) (-44.6327, -10.7848) knots 0 0 0 0 1 1 1 1
  spline S607 degree 3 poles (-44.6327, -10.7848) (-44.6381, -10.9862) (-44.6577, -11.1582) (-44.7266, -11.35) knots 0 0 0 0 1 1 1 1
  spline S608 degree 3 poles (-44.7266, -11.35) (-44.9081, -11.3566) (-45.0537, -11.313) (-45.2258, -11.2573) knots 0 0 0 0 1 1 1 1
  spline S609 degree 3 poles (-45.2258, -11.2573) (-45.439, -11.1904) (-45.6418, -11.1455) (-45.8645, -11.1268) knots 0 0 0 0 1 1 1 1
  spline S610 degree 3 poles (-45.8645, -11.1268) (-45.9778, -11.1127) (-46.0814, -11.0846) (-46.1912, -11.0532) knots 0 0 0 0 1 1 1 1
  spline S611 degree 3 poles (-46.1912, -11.0532) (-46.9827, -10.842) (-47.8002, -10.9782) (-48.5992, -11.0739) knots 0 0 0 0 1 1 1 1
  spline S612 degree 3 poles (-48.5992, -11.0739) (-48.9126, -11.1105) (-49.223, -11.1322) (-49.5383, -11.143) knots 0 0 0 0 1 1 1 1
  spline S613 degree 3 poles (-49.5383, -11.143) (-49.7136, -11.1505) (-49.8862, -11.168) (-50.0601, -11.1906) knots 0 0 0 0 1 1 1 1
  spline S614 degree 3 poles (-50.0601, -11.1906) (-50.0902, -11.1943) (-50.1202, -11.198) (-50.1512, -11.2018) knots 0 0 0 0 1 1 1 1
  spline S615 degree 3 poles (-50.1512, -11.2018) (-50.2227, -11.2107) (-50.2942, -11.2198) (-50.3657, -11.229) knots 0 0 0 0 1 1 1 1
  spline S616 degree 3 poles (-50.3657, -11.229) (-50.3681, -11.2158) (-50.3704, -11.2026) (-50.3728, -11.189) knots 0 0 0 0 1 1 1 1
  line L4 (-50.8593, 14.9966) -> (-50.9465, 15.0225)
  line L5 (-50.7862, 15.0507) -> (-50.8734, 15.0767)
  spline S617 degree 3 poles (-37.2216, 13.6788) (-37.21, 13.7302) (-37.21, 13.7302) (-37.1981, 13.7827) knots 0 0 0 0 1 1 1 1
  spline S618 degree 3 poles (-37.1981, 13.7827) (-37.1896, 13.8198) (-37.181, 13.8569) (-37.1722, 13.8952) knots 0 0 0 0 1 1 1 1
  spline S619 degree 3 poles (-37.1722, 13.8952) (-37.1635, 13.9331) (-37.1548, 13.9711) (-37.1459, 14.0103) knots 0 0 0 0 1 1 1 1
  spline S620 degree 3 poles (-37.1459, 14.0103) (-37.1274, 14.0907) (-37.1089, 14.1711) (-37.0902, 14.2514) knots 0 0 0 0 1 1 1 1
  spline S621 degree 3 poles (-37.0902, 14.2514) (-37.0617, 14.3748) (-37.0337, 14.4983) (-37.0057, 14.6218) knots 0 0 0 0 1 1 1 1
  spline S622 degree 3 poles (-37.0057, 14.6218) (-36.9877, 14.6998) (-36.9697, 14.7777) (-36.9517, 14.8557) knots 0 0 0 0 1 1 1 1
  spline S623 degree 3 poles (-36.9517, 14.8557) (-36.9433, 14.8928) (-36.935, 14.93) (-36.9263, 14.9683) knots 0 0 0 0 1 1 1 1
  spline S624 degree 3 poles (-36.9263, 14.9683) (-36.9183, 15.0025) (-36.9103, 15.0367) (-36.902, 15.072) knots 0 0 0 0 1 1 1 1
  spline S625 degree 3 poles (-36.902, 15.072) (-36.8951, 15.1022) (-36.8881, 15.1324) (-36.8809, 15.1636) knots 0 0 0 0 1 1 1 1
  spline S626 degree 3 poles (-36.8809, 15.1636) (-36.8622, 15.2419) (-36.8622, 15.2419) (-36.7839, 15.2892) knots 0 0 0 0 1 1 1 1
  spline S627 degree 3 poles (-36.7839, 15.2892) (-36.6879, 15.1942) (-36.592, 15.0993) (-36.4961, 15.0043) knots 0 0 0 0 1 1 1 1
  spline S628 degree 3 poles (-36.4961, 15.0043) (-36.4692, 14.9776) (-36.4422, 14.951) (-36.4144, 14.9235) knots 0 0 0 0 1 1 1 1
  spline S629 degree 3 poles (-36.4144, 14.9235) (-36.3371, 14.8468) (-36.26, 14.7699) (-36.183, 14.6929) knots 0 0 0 0 1 1 1 1
  spline S630 degree 3 poles (-36.183, 14.6929) (-36.1618, 14.6718) (-36.1406, 14.6507) (-36.1188, 14.6289) knots 0 0 0 0 1 1 1 1
  spline S631 degree 3 poles (-36.1188, 14.6289) (-36.0149, 14.5305) (-36.0149, 14.5305) (-35.9663, 14.4006) knots 0 0 0 0 1 1 1 1
  spline S632 degree 3 poles (-35.9663, 14.4006) (-36.1126, 14.2888) (-36.259, 14.1771) (-36.4053, 14.0653) knots 0 0 0 0 1 1 1 1
  spline S633 degree 3 poles (-36.4053, 14.0653) (-36.4551, 14.0273) (-36.5048, 13.9894) (-36.5545, 13.9514) knots 0 0 0 0 1 1 1 1
  spline S634 degree 3 poles (-36.5545, 13.9514) (-36.6262, 13.8966) (-36.698, 13.8418) (-36.7697, 13.787) knots 0 0 0 0 1 1 1 1
  spline S635 degree 3 poles (-36.7697, 13.787) (-36.7917, 13.7702) (-36.8137, 13.7534) (-36.8363, 13.7361) knots 0 0 0 0 1 1 1 1
  spline S636 degree 3 poles (-36.8363, 13.7361) (-36.9705, 13.6337) (-37.1055, 13.5326) (-37.2413, 13.4323) knots 0 0 0 0 1 1 1 1
  spline S637 degree 3 poles (-37.2413, 13.4323) (-37.2579, 13.5266) (-37.2428, 13.5855) (-37.2216, 13.6788) knots 0 0 0 0 1 1 1 1
  spline S638 degree 3 poles (-29.2882, 12.6041) (-28.8697, 12.7557) (-28.5896, 12.7131) (-28.1934, 12.5283) knots 0 0 0 0 1 1 1 1
  spline S639 degree 3 poles (-28.1934, 12.5283) (-28.0851, 12.4763) (-27.9778, 12.4225) (-27.8706, 12.3684) knots 0 0 0 0 1 1 1 1
  spline S640 degree 3 poles (-27.8706, 12.3684) (-27.7226, 12.2949) (-27.5716, 12.228) (-27.4211, 12.1599) knots 0 0 0 0 1 1 1 1
  spline S641 degree 3 poles (-27.4211, 12.1599) (-27.3957, 12.147) (-27.3703, 12.134) (-27.3442, 12.1207) knots 0 0 0 0 1 1 1 1
  spline S642 degree 3 poles (-27.3442, 12.1207) (-27.3418, 12.1075) (-27.3395, 12.0943) (-27.3371, 12.0806) knots 0 0 0 0 1 1 1 1
  spline S643 degree 3 poles (-27.3371, 12.0806) (-27.3612, 12.0758) (-27.3853, 12.071) (-27.4102, 12.0661) knots 0 0 0 0 1 1 1 1
  spline S644 degree 3 poles (-27.4102, 12.0661) (-27.6928, 11.9997) (-27.879, 11.8794) (-28.1005, 11.6956) knots 0 0 0 0 1 1 1 1
  spline S645 degree 3 poles (-28.1005, 11.6956) (-28.1317, 11.6706) (-28.1628, 11.6456) (-28.1949, 11.6198) knots 0 0 0 0 1 1 1 1
  spline S646 degree 3 poles (-28.1949, 11.6198) (-28.2708, 11.5588) (-28.3462, 11.4972) (-28.4212, 11.4351) knots 0 0 0 0 1 1 1 1
  spline S647 degree 3 poles (-28.4212, 11.4351) (-28.5203, 11.5389) (-28.5593, 11.6131) (-28.6197, 11.7409) knots 0 0 0 0 1 1 1 1
  spline S648 degree 3 poles (-28.6197, 11.7409) (-28.7463, 11.9829) (-28.9129, 12.1609) (-29.1051, 12.3513) knots 0 0 0 0 1 1 1 1
  spline S649 degree 3 poles (-29.1051, 12.3513) (-29.2274, 12.4594) (-29.2274, 12.4594) (-29.2882, 12.6041) knots 0 0 0 0 1 1 1 1
  spline S650 degree 3 poles (-20.2846, -8.9403) (-19.8892, -8.8299) (-19.4907, -8.7519) (-19.0871, -8.6784) knots 0 0 0 0 1 1 1 1
  spline S651 degree 3 poles (-19.0871, -8.6784) (-18.9719, -8.6574) (-18.8567, -8.6361) (-18.7416, -8.6149) knots 0 0 0 0 1 1 1 1
  spline S652 degree 3 poles (-18.7416, -8.6149) (-18.5768, -8.5844) (-18.4119, -8.554) (-18.2471, -8.5237) knots 0 0 0 0 1 1 1 1
  spline S653 degree 3 poles (-18.2471, -8.5237) (-16.8732, -8.2708) (-15.5027, -8.0084) (-14.1374, -7.713) knots 0 0 0 0 1 1 1 1
  spline S654 degree 3 poles (-14.1374, -7.713) (-13.5391, -7.5836) (-12.9449, -7.4619) (-12.3336, -7.4144) knots 0 0 0 0 1 1 1 1
  spline S655 degree 3 poles (-12.3336, -7.4144) (-12.4282, -7.5573) (-12.5326, -7.677) (-12.6531, -7.7987) knots 0 0 0 0 1 1 1 1
  spline S656 degree 3 poles (-12.6531, -7.7987) (-12.7577, -7.9044) (-12.8551, -8.008) (-12.9472, -8.125) knots 0 0 0 0 1 1 1 1
  spline S657 degree 3 poles (-12.9472, -8.125) (-13.0634, -8.2533) (-13.1826, -8.3271) (-13.3333, -8.4065) knots 0 0 0 0 1 1 1 1
  spline S658 degree 3 poles (-13.3333, -8.4065) (-13.9324, -8.7442) (-14.363, -9.2406) (-14.813, -9.7517) knots 0 0 0 0 1 1 1 1
  spline S659 degree 3 poles (-14.813, -9.7517) (-14.9284, -9.8819) (-15.0445, -10.0109) (-15.1642, -10.1372) knots 0 0 0 0 1 1 1 1
  spline S660 degree 3 poles (-15.1642, -10.1372) (-15.2631, -10.2442) (-15.2631, -10.2442) (-15.3414, -10.3514) knots 0 0 0 0 1 1 1 1
  spline S661 degree 3 poles (-15.3414, -10.3514) (-15.432, -10.4604) (-15.4865, -10.5096) (-15.6214, -10.5552) knots 0 0 0 0 1 1 1 1
  spline S662 degree 3 poles (-15.6214, -10.5552) (-15.8636, -10.5279) (-16.0834, -10.4521) (-16.3132, -10.3731) knots 0 0 0 0 1 1 1 1
  spline S663 degree 3 poles (-16.3132, -10.3731) (-16.4601, -10.3242) (-16.608, -10.2803) (-16.7567, -10.2374) knots 0 0 0 0 1 1 1 1
  spline S664 degree 3 poles (-16.7567, -10.2374) (-17.417, -10.0467) (-18.0716, -9.8426) (-18.72, -9.6145) knots 0 0 0 0 1 1 1 1
  spline S665 degree 3 poles (-18.72, -9.6145) (-18.7568, -9.6016) (-18.7936, -9.5888) (-18.8315, -9.5755) knots 0 0 0 0 1 1 1 1
  spline S666 degree 3 poles (-18.8315, -9.5755) (-19.207, -9.4434) (-19.5785, -9.3047) (-19.9437, -9.1461) knots 0 0 0 0 1 1 1 1
  spline S667 degree 3 poles (-19.9437, -9.1461) (-19.9721, -9.1339) (-20.0004, -9.1216) (-20.0296, -9.109) knots 0 0 0 0 1 1 1 1
  spline S668 degree 3 poles (-20.0296, -9.109) (-20.1747, -9.0482) (-20.1747, -9.0482) (-20.2846, -8.9403) knots 0 0 0 0 1 1 1 1
  spline S669 degree 3 poles (-8.3515, -3.8776) (-8.3386, -3.8501) (-8.3257, -3.8226) (-8.3125, -3.7942) knots 0 0 0 0 1 1 1 1
  spline S670 degree 3 poles (-8.3125, -3.7942) (-8.2806, -3.7262) (-8.2484, -3.6583) (-8.2162, -3.5904) knots 0 0 0 0 1 1 1 1
  spline S671 degree 3 poles (-8.2162, -3.5904) (-8.1894, -3.6266) (-8.1894, -3.6266) (-8.1621, -3.6635) knots 0 0 0 0 1 1 1 1
  spline S672 degree 3 poles (-8.1621, -3.6635) (-8.1884, -3.7667) (-8.1884, -3.7667) (-8.2348, -3.8803) knots 0 0 0 0 1 1 1 1
  spline S673 degree 3 poles (-8.2348, -3.8803) (-8.2495, -3.919) (-8.2641, -3.9577) (-8.2792, -3.9976) knots 0 0 0 0 1 1 1 1
  spline S674 degree 3 poles (-8.2792, -3.9976) (-8.3311, -4.105) (-8.3848, -4.1735) (-8.4708, -4.2549) knots 0 0 0 0 1 1 1 1
  spline S675 degree 3 poles (-8.4708, -4.2549) (-8.495, -4.1179) (-8.4095, -3.9996) (-8.3515, -3.8776) knots 0 0 0 0 1 1 1 1
  spline S676 degree 3 poles (-81.6891, -16.5457) (-81.522, -16.9771) (-81.2873, -17.3601) (-80.8833, -17.6015) knots 0 0 0 0 1 1 1 1
  spline S677 degree 3 poles (-80.8833, -17.6015) (-80.839, -17.6209) (-80.7947, -17.6404) (-80.749, -17.6604) knots 0 0 0 0 1 1 1 1
  spline S678 degree 3 poles (-80.749, -17.6604) (-80.7576, -17.6892) (-80.7661, -17.718) (-80.7749, -17.7476) knots 0 0 0 0 1 1 1 1
  spline S679 degree 3 poles (-80.7749, -17.7476) (-80.7547, -18.1502) (-80.733, -18.5132) (-80.4411, -18.8147) knots 0 0 0 0 1 1 1 1
  spline S680 degree 3 poles (-80.4411, -18.8147) (-80.1666, -19.0557) (-79.8231, -19.2792) (-79.4465, -19.2629) knots 0 0 0 0 1 1 1 1
  spline S681 degree 3 poles (-79.4465, -19.2629) (-79.078, -19.2204) (-78.7212, -19.1324) (-78.3669, -19.0253) knots 0 0 0 0 1 1 1 1
  spline S682 degree 3 poles (-78.3669, -19.0253) (-78.2238, -18.9854) (-78.0786, -18.9598) (-77.9323, -18.9348) knots 0 0 0 0 1 1 1 1
  spline S683 degree 3 poles (-77.9323, -18.9348) (-77.9031, -18.9295) (-77.874, -18.9242) (-77.844, -18.9187) knots 0 0 0 0 1 1 1 1
  spline S684 degree 3 poles (-77.844, -18.9187) (-77.6914, -18.8921) (-77.5482, -18.8756) (-77.3935, -18.8863) knots 0 0 0 0 1 1 1 1
  spline S685 degree 3 poles (-77.3935, -18.8863) (-77.3615, -18.9522) (-77.3615, -18.9522) (-77.3287, -19.0194) knots 0 0 0 0 1 1 1 1
  spline S686 degree 3 poles (-77.3287, -19.0194) (-77.1747, -19.3032) (-76.9737, -19.5557) (-76.7763, -19.8101) knots 0 0 0 0 1 1 1 1
  spline S687 degree 3 poles (-76.7763, -19.8101) (-76.75, -19.844) (-76.75, -19.844) (-76.7233, -19.8785) knots 0 0 0 0 1 1 1 1
  spline S688 degree 3 poles (-76.7233, -19.8785) (-75.9161, -20.9118) (-74.8767, -21.4669) (-73.5922, -21.6603) knots 0 0 0 0 1 1 1 1
  spline S689 degree 3 poles (-73.5922, -21.6603) (-73.422, -21.6579) (-73.3291, -21.6198) (-73.1781, -21.5496) knots 0 0 0 0 1 1 1 1
  spline S690 degree 3 poles (-73.1781, -21.5496) (-73.0555, -21.5013) (-72.9383, -21.4927) (-72.8079, -21.4808) knots 0 0 0 0 1 1 1 1
  spline S691 degree 3 poles (-72.8079, -21.4808) (-72.539, -21.4538) (-72.3239, -21.422) (-72.1452, -21.2067) knots 0 0 0 0 1 1 1 1
  spline S692 degree 3 poles (-72.1452, -21.2067) (-72.0643, -21.0928) (-71.9942, -20.9757) (-71.9244, -20.8547) knots 0 0 0 0 1 1 1 1
  spline S693 degree 3 poles (-71.9244, -20.8547) (-71.8979, -20.816) (-71.8714, -20.7772) (-71.8441, -20.7373) knots 0 0 0 0 1 1 1 1
  spline S694 degree 3 poles (-71.8441, -20.7373) (-71.6479, -20.448) (-71.5209, -20.1421) (-71.4058, -19.8132) knots 0 0 0 0 1 1 1 1
  spline S695 degree 3 poles (-71.4058, -19.8132) (-71.3881, -19.7647) (-71.3704, -19.7161) (-71.3522, -19.6661) knots 0 0 0 0 1 1 1 1
  spline S696 degree 3 poles (-71.3522, -19.6661) (-71.0872, -18.8933) (-70.9324, -17.9595) (-71.0496, -17.148) knots 0 0 0 0 1 1 1 1
  spline S697 degree 3 poles (-71.0496, -17.148) (-71.053, -17.1157) (-71.0565, -17.0833) (-71.0601, -17.05) knots 0 0 0 0 1 1 1 1
  spline S698 degree 3 poles (-71.0601, -17.05) (-71.0721, -16.9601) (-71.0909, -16.8754) (-71.1132, -16.7875) knots 0 0 0 0 1 1 1 1
  spline S699 degree 3 poles (-71.1132, -16.7875) (-71.1245, -16.7417) (-71.1359, -16.6959) (-71.1476, -16.6487) knots 0 0 0 0 1 1 1 1
  spline S700 degree 3 poles (-71.1476, -16.6487) (-71.3454, -15.9048) (-71.7007, -15.2349) (-72.1136, -14.5894) knots 0 0 0 0 1 1 1 1
  spline S701 degree 3 poles (-72.1136, -14.5894) (-72.1379, -14.5508) (-72.1622, -14.5121) (-72.1873, -14.4723) knots 0 0 0 0 1 1 1 1
  spline S702 degree 3 poles (-72.1873, -14.4723) (-72.2092, -14.4383) (-72.2312, -14.4043) (-72.2538, -14.3693) knots 0 0 0 0 1 1 1 1
  spline S703 degree 3 poles (-72.2538, -14.3693) (-72.3331, -14.2016) (-72.3068, -14.0968) (-72.2497, -13.9231) knots 0 0 0 0 1 1 1 1
  spline S704 degree 3 poles (-72.2497, -13.9231) (-72.2289, -13.8683) (-72.208, -13.8136) (-72.1869, -13.7589) knots 0 0 0 0 1 1 1 1
  spline S705 degree 3 poles (-72.1869, -13.7589) (-72.022, -13.31) (-71.9152, -12.8483) (-71.8045, -12.3837) knots 0 0 0 0 1 1 1 1
  spline S706 degree 3 poles (-71.8045, -12.3837) (-71.5918, -11.3454) (-71.5918, -11.3454) (-71.112, -10.4212) knots 0 0 0 0 1 1 1 1
  spline S707 degree 3 poles (-71.112, -10.4212) (-70.9637, -10.2157) (-70.8652, -9.9793) (-70.7586, -9.7505) knots 0 0 0 0 1 1 1 1
  spline S708 degree 3 poles (-70.7586, -9.7505) (-70.7429, -9.7167) (-70.7271, -9.6829) (-70.7109, -9.648) knots 0 0 0 0 1 1 1 1
  spline S709 degree 3 poles (-70.7109, -9.648) (-70.697, -9.6177) (-70.6831, -9.5874) (-70.6688, -9.5562) knots 0 0 0 0 1 1 1 1
  spline S710 degree 3 poles (-70.6688, -9.5562) (-70.6287, -9.4715) (-70.6287, -9.4715) (-70.5711, -9.3963) knots 0 0 0 0 1 1 1 1
  spline S711 degree 3 poles (-70.5711, -9.3963) (-70.5277, -9.3316) (-70.5277, -9.3316) (-70.5418, -9.2515) knots 0 0 0 0 1 1 1 1
  spline S712 degree 3 poles (-70.5418, -9.2515) (-70.5206, -9.2367) (-70.4993, -9.2218) (-70.4775, -9.2066) knots 0 0 0 0 1 1 1 1
  spline S713 degree 3 poles (-70.4775, -9.2066) (-70.3957, -9.1431) (-70.3957, -9.1431) (-70.3396, -9.0661) knots 0 0 0 0 1 1 1 1
  spline S714 degree 3 poles (-70.3396, -9.0661) (-70.208, -8.9528) (-70.0673, -8.9356) (-69.8961, -8.9311) knots 0 0 0 0 1 1 1 1
  spline S715 degree 3 poles (-69.8961, -8.9311) (-69.7484, -8.9627) (-69.6142, -9.0175) (-69.4755, -9.0764) knots 0 0 0 0 1 1 1 1
  spline S716 degree 3 poles (-69.4755, -9.0764) (-69.4174, -9.0999) (-69.4174, -9.0999) (-69.3581, -9.1238) knots 0 0 0 0 1 1 1 1
  spline S717 degree 3 poles (-69.3581, -9.1238) (-69.2416, -9.1715) (-69.1258, -9.2207) (-69.0101, -9.2705) knots 0 0 0 0 1 1 1 1
  spline S718 degree 3 poles (-69.0101, -9.2705) (-68.9778, -9.2845) (-68.9455, -9.2984) (-68.9123, -9.3127) knots 0 0 0 0 1 1 1 1
  spline S719 degree 3 poles (-68.9123, -9.3127) (-68.7034, -9.4039) (-68.4972, -9.5002) (-68.2914, -9.5982) knots 0 0 0 0 1 1 1 1
  spline S720 degree 3 poles (-68.2914, -9.5982) (-68.2578, -9.6141) (-68.2242, -9.6299) (-68.1896, -9.6463) knots 0 0 0 0 1 1 1 1
  spline S721 degree 3 poles (-68.1896, -9.6463) (-67.6441, -9.9044) (-67.118, -10.1813) (-66.6043, -10.4986) knots 0 0 0 0 1 1 1 1
  spline S722 degree 3 poles (-66.6043, -10.4986) (-66.6644, -10.7656) (-66.7653, -10.938) (-66.9267, -11.1573) knots 0 0 0 0 1 1 1 1
  spline S723 degree 3 poles (-66.9267, -11.1573) (-67.2044, -11.5623) (-67.382, -11.9789) (-67.2931, -12.4694) knots 0 0 0 0 1 1 1 1
  spline S724 degree 3 poles (-67.2931, -12.4694) (-67.288, -12.4964) (-67.2829, -12.5233) (-67.2776, -12.551) knots 0 0 0 0 1 1 1 1
  spline S725 degree 3 poles (-67.2776, -12.551) (-67.2726, -12.5788) (-67.2675, -12.6065) (-67.2623, -12.635) knots 0 0 0 0 1 1 1 1
  spline S726 degree 3 poles (-67.2623, -12.635) (-67.2498, -12.7029) (-67.2371, -12.7707) (-67.2244, -12.8385) knots 0 0 0 0 1 1 1 1
  spline S727 degree 3 poles (-67.2244, -12.8385) (-67.2715, -12.847) (-67.2715, -12.847) (-67.3196, -12.8556) knots 0 0 0 0 1 1 1 1
  spline S728 degree 3 poles (-67.3196, -12.8556) (-67.5691, -12.9092) (-67.7478, -12.955) (-67.8952, -13.1721) knots 0 0 0 0 1 1 1 1
  spline S729 degree 3 poles (-67.8952, -13.1721) (-68.0384, -13.4562) (-68.008, -13.7359) (-67.9221, -14.0355) knots 0 0 0 0 1 1 1 1
  spline S730 degree 3 poles (-67.9221, -14.0355) (-67.7936, -14.3559) (-67.5493, -14.5382) (-67.243, -14.68) knots 0 0 0 0 1 1 1 1
  spline S731 degree 3 poles (-67.243, -14.68) (-66.895, -14.817) (-66.5226, -14.8647) (-66.1548, -14.9218) knots 0 0 0 0 1 1 1 1
  spline S732 degree 3 poles (-66.1548, -14.9218) (-66.1791, -14.9265) (-66.2035, -14.9312) (-66.2285, -14.936) knots 0 0 0 0 1 1 1 1
  spline S733 degree 3 poles (-66.2285, -14.936) (-67.3248, -15.1512) (-67.3248, -15.1512) (-67.6589, -15.6087) knots 0 0 0 0 1 1 1 1
  spline S734 degree 3 poles (-67.6589, -15.6087) (-67.789, -15.8112) (-67.8474, -15.9667) (-67.8281, -16.2082) knots 0 0 0 0 1 1 1 1
  spline S735 degree 3 poles (-67.8281, -16.2082) (-67.8501, -16.2196) (-67.872, -16.231) (-67.8946, -16.2427) knots 0 0 0 0 1 1 1 1
  spline S736 degree 3 poles (-67.8946, -16.2427) (-67.9864, -16.2912) (-68.0769, -16.3415) (-68.1675, -16.392) knots 0 0 0 0 1 1 1 1
  spline S737 degree 3 poles (-68.1675, -16.392) (-68.208, -16.4136) (-68.2484, -16.4353) (-68.2902, -16.4575) knots 0 0 0 0 1 1 1 1
  spline S738 degree 3 poles (-68.2902, -16.4575) (-68.5614, -16.7304) (-68.5415, -17.1913) (-68.5715, -17.5543) knots 0 0 0 0 1 1 1 1
  spline S739 degree 3 poles (-68.5715, -17.5543) (-68.5864, -17.7278) (-68.6122, -17.8968) (-68.6412, -18.0684) knots 0 0 0 0 1 1 1 1